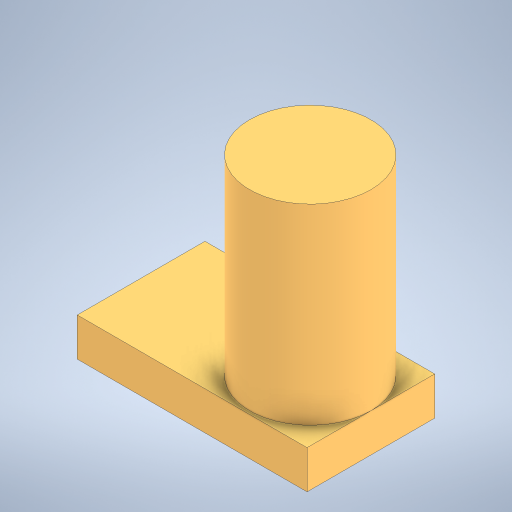
# Autodesk Inventor part: Candado
Saved by Autodesk Inventor 2024 (Build 280153000, 153)
## iProperties
Created: 2024-04-23
Part Number: Candado
Material: Generic
Document SubType Name: Modeling
Designer: samue
Density: 1 g/cm^3
Appearance: Default
Author: samue
Autodesk Inventor part; units mm, degrees
ref_plane "YZ Plane" through (0, 0, 0) normal (1, 0, 0) x (0, 1, 0)
ref_plane "XZ Plane" through (0, 0, 0) normal (0, 1, 0) x (-1, 0, 0)
ref_plane "XY Plane" through (0, 0, 0) normal (0, 0, 1) x (1, 0, 0)
sketch "Sketch1" plane through (0, 0, 0) normal (0, 1, 0) x (-1, 0, 0)
  line L0 (9, 5) -> (-9, 5)
  line L1 (-9, 5) -> (-9, -5)
  line L2 (-9, -5) -> (9, -5)
  line L3 (9, -5) -> (9, 5)
  line L4 (9, 5) -> (-9, -5) construction
  line L5 (-9, 5) -> (9, -5) construction
  point P0 (0, 0)
  dimension "d0" = 18
  dimension "d1" = 10
  constraints: 12 end point, 2 midpoint, 2 parallel, 1 horizontal, 1 perpendicular
  measures "d0" distance of L2.end L1.end
  measures "d1" distance of L1.end L0.end
extrude "Extrusion1" add sketch "Sketch1" along normal blind 3
sketch "Sketch2" plane through (0, 3, 0) normal (0, 1, 0) x (1, 0, 0)
  circle A0 centre (4.25, 0) radius 4.75
  line L0 (9, -5) -> (9, 5) projected
  point P0 (0, 0)
  dimension "d4" = 9.5
  constraints: 1 centre point, 1 tangent
  measures "d4" diameter of A0
extrude "Extrusion2" add sketch "Sketch2" along normal blind 15
body "Solid1"
